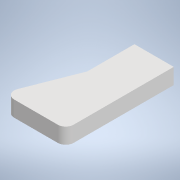
# Autodesk Inventor part: footbtn
Saved by Autodesk Inventor 2022 (Build 260153000, 153)
## iProperties
Created: 2025-06-24
Part Number: footbtn
Material: Типовые
Document SubType Name: Modeling
Designer: korsh524
Density: 1 g/cm^3
Appearance: По умолчанию
Author: korsh524
Autodesk Inventor part; units mm, degrees
ref_plane "YZ Plane" through (0, 0, 0) normal (1, 0, 0) x (0, 1, 0)
ref_plane "XZ Plane" through (0, 0, 0) normal (0, 1, 0) x (-1, 0, 0)
ref_plane "XY Plane" through (0, 0, 0) normal (0, 0, 1) x (1, 0, 0)
sketch "Эскиз1" plane through (0, 0, 0) normal (0, 0, 1) x (1, 0, 0)
  line L0 (-25, -12.5) -> (-25, -8.5) projected
  line L1 (-15, -12.5) -> (-25, -12.5) projected
  line L2 (-25, -8.5) -> (-15, -8.5) projected
  line L3 (-15, -8.5) -> (-15, -12.5) projected
  point P0 (0, 0)
extrude "Выдавливание1" add sketch "Эскиз1" against normal blind 12
sketch "Эскиз2" plane through (-25, -8.5, 0) normal (0, 1, 0) x (1, 0, 0)
  line L0 (-6.047, -15.4734) -> (10, -15.4734)
  line L1 (10, -15.4734) -> (10, 0)
  line L2 (0, 0) -> (10, 0) projected
  line L3 (0, 0) -> (-6.047, -15.4734)
  line L4 (0, 0) -> (10, 0)
  point P0 (25, 0)
  constraints: 8 end point, 2 horizontal, 1 perpendicular
extrude "Выдавливание2" add sketch "Эскиз2" against normal blind 4
fillet "Сопряжение1" radius 2 2 edges at (-15, -10.5, 15.4734) (-31.047, -10.5, 15.4734)
